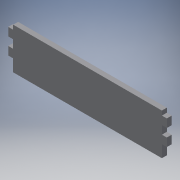
# Autodesk Inventor part: мальенькое дно 2
Saved by Autodesk Inventor 2019 (Build 230136000, 136)
## iProperties
Created: 2022-02-24
Part Number: мальенькое дно 2
Material: Типовые
Document SubType Name: Modeling
Designer: korsh
Density: 1 g/cm^3
Appearance: По умолчанию
Author: korsh
Autodesk Inventor part; units mm, degrees
ref_plane "YZ Plane" through (0, 0, 0) normal (1, 0, 0) x (0, 1, 0)
ref_plane "XZ Plane" through (0, 0, 0) normal (0, 1, 0) x (-1, 0, 0)
ref_plane "XY Plane" through (0, 0, 0) normal (0, 0, 1) x (1, 0, 0)
sketch "Эскиз1" plane through (0, 0, 0) normal (0, 0, 1) x (1, 0, 0)
  line L0 (0, 0) -> (0, -10) projected
  line L1 (0, 0) -> (-6, 0) projected
  line L2 (-6, -10) -> (-6, 0) projected
  line L3 (0, -10) -> (-6, -10) projected
  line L4 (0, -20) -> (0, -30) projected
  line L5 (0, -20) -> (-6, -20) projected
  line L6 (-6, -30) -> (-6, -20) projected
  line L7 (0, -30) -> (-6, -30) projected
  line L8 (0, -37.8173) -> (0, -44.6471) projected
  line L9 (0, -37.8173) -> (-6, -37.8173) projected
  line L10 (-6, -44.6471) -> (-6, -37.8173) projected
  line L11 (0, -44.6471) -> (-6, -44.6471) projected
  line L12 (-6, 0) -> (-6, 5.2722) projected
  line L13 (-6, -38.785) -> (-6, -30) projected
  line L14 (-186, 0) -> (-186, -10) projected
  line L15 (-186, 0) -> (-192, 0) projected
  line L16 (-192, -10) -> (-192, 0) projected
  line L17 (-186, -10) -> (-192, -10) projected
  line L18 (-186, -20) -> (-186, -30) projected
  line L19 (-186, -20) -> (-192, -20) projected
  line L20 (-192, -30) -> (-192, -20) projected
  line L21 (-186, -30) -> (-192, -30) projected
  line L22 (-186, -30) -> (-186, -38.785) projected
  line L23 (-186, 9.4324) -> (-186, 5.2722) projected
  line L24 (-6, -44.6471) -> (-186, -44.6471)
  line L25 (-186, -44.6471) -> (-186, 5.2722)
  line L26 (-186, 5.2722) -> (-6, 5.2722)
  line L27 (-6, 5.2722) -> (-6, -44.6471)
  constraints: 8 end point, 2 parallel, 1 horizontal, 1 perpendicular
extrude "Выдавливание1" add sketch "Эскиз1" along normal blind 6 contours L0 L3 L2 L1 | L2 L27 L6 L13 L10 L24 L25 L22 L18 L14 L26 L12 | L5 L4 L7 L6 | L14 L17 L16 L15 | L18 L21 L20 L19
sketch "Эскиз3" plane through (0, 0, 6) normal (0, 0, 1) x (1, 0, 0)
  line L0 (-186, 0) -> (-192, 0) projected
  line L1 (-192, 0) -> (-192, -10) projected
  line L2 (-192, -10) -> (-186, -10) projected
  line L3 (-186, -10) -> (-186, -20) projected
  line L4 (-186, -20) -> (-192, -20) projected
  line L5 (-192, -20) -> (-192, -30) projected
  line L6 (-192, -30) -> (-186, -30) projected
  line L7 (-186, -30) -> (-186, -44.6471) projected
  line L8 (-186, -44.6471) -> (-6, -44.6471) projected
  line L9 (-6, -44.6471) -> (-6, -30) projected
  line L10 (-6, -30) -> (0, -30) projected
  line L11 (0, -30) -> (0, -20) projected
  line L12 (0, -20) -> (-6, -20) projected
  line L13 (-6, -20) -> (-6, -10) projected
  line L14 (-6, -10) -> (0, -10) projected
  line L15 (0, -10) -> (0, 0) projected
  line L16 (0, 0) -> (-6, 0) projected
  line L17 (-6, 0) -> (-6, 5.2722) projected
  line L18 (-6, 5.2722) -> (-186, 5.2722) projected
  line L19 (-186, 5.2722) -> (-186, 0) projected
  line L20 (-6, -38.785) -> (0, -38.785) projected
  line L21 (-192, -38.785) -> (-186, -38.785) projected
  line L22 (-186, -44.6471) -> (-6, -44.6471) projected
  line L23 (-6, -44.6471) -> (-186, -44.6471)
  line L24 (-186, -44.6471) -> (-186, -38.785)
  line L25 (-186, -38.785) -> (-6, -38.785)
  line L26 (-6, -38.785) -> (-6, -44.6471)
  constraints: 8 end point, 2 parallel, 1 horizontal, 1 perpendicular
extrude "Выдавливание2" cut sketch "Эскиз3" against normal blind 6 contours L25 L9 L8 L7
